Autodesk Inventor part; units mm, degrees
(part 2 of 2)
extrude "Extrusion65" cut sketch "Sketch70" against normal blind 1.5 contours L6 L7 L8 L0 | L4 L17 L14 L15
sketch "Sketch71" plane through (0, 1.5, 0) normal (0, 1, 0) x (1, 0, 0)
  line L0 (6.4642, -4.9) -> (13.4642, -4.9) projected
  line L1 (-3.6078, -4.9) -> (3.3922, -4.9) projected
  line L2 (-3.6078, -3.9) -> (3.3922, -3.9)
  line L3 (6.4642, -3.9) -> (13.4642, -3.9)
  line L4 (-3.4042, -4.9) -> (3.3922, -4.9)
  line L5 (13.4642, -4.9) -> (6.4642, -4.9)
  line L6 (6.4642, -4.9) -> (6.4642, -3.9)
  line L7 (13.4642, -4.9) -> (13.4642, -3.9)
  line L8 (6.4642, -4.9) -> (6.4642, -3.9)
  line L9 (13.4642, -4.9) -> (6.4642, -4.9)
  line L10 (3.3922, -3.9) -> (3.3922, -4.9)
  line L11 (3.3922, -4.9) -> (-3.6078, -4.9)
  line L12 (-3.6078, -4.9) -> (-3.6078, -3.9)
  point P0 (3.3922, -22.9)
  point P1 (0, 0)
  dimension "d349" = 7
  dimension "d351" = 7
  constraints: 22 end point, 4 collinear, 1 point on line
  measures "d349" distance of L2.start L2.end
  measures "d351" distance of L3.start L3.end
extrude "Extrusion66" cut sketch "Sketch71" against normal blind 1.5
sketch "Sketch75" plane through (0, 1.5, 0) normal (0, 1, 0) x (1, 0, 0)
  line L0 (-14, 20) -> (14, 20) projected
  line L1 (-14, 20) -> (0, 20)
  line L2 (0, 20) -> (0, 11.7)
  line L3 (0, 11.7) -> (-11.6, 11.7)
  line L4 (-11.6, 11.7) -> (12, 11.7)
  line L5 (12, 11.7) -> (12, -0.7)
  line L6 (12, -0.7) -> (-11.6, -0.7)
  line L7 (-11.6, -0.7) -> (-11.6, 11.7)
  point P0 (0, 0)
  dimension "d359" = 8.3
  dimension "d360" = 11.6
  dimension "d361" = 23.6
  dimension "d362" = 12.4
  constraints: 14 end point, 3 perpendicular, 2 parallel, 1 horizontal, 1 midpoint
  measures "d359" distance of L1.end L2.end
  measures "d360" distance of L2.end L3.end
  measures "d361" distance of L5.end L6.end
  measures "d362" distance of L4.end L5.end
extrude "Extrusion67" cut sketch "Sketch75" against normal blind 1.5
sketch "Sketch76" plane through (0, 1.5, 0) normal (0, 1, 0) x (1, 0, 0)
  line L0 (-11.6, -0.7) -> (-11.6, 11.7) projected
  circle A0 centre (13.95, 5.5) radius 1.5 projected
  circle A1 centre (-13.95, 5.5) radius 1.5 projected
  line L1 (6.4642, -3.9) -> (13.4642, -3.9) projected
  line L2 (-13.95, 5.5) -> (13.95, 5.5)
  line L3 (-11.6, 11.7) -> (-12, 11.7)
  line L4 (-12, 11.7) -> (-12, -0.7)
  line L5 (-12, -0.7) -> (-11.6, -0.7)
  line L6 (-11.6, 11.7) -> (-11.6, -0.7)
  point P0 (0, 0)
  dimension "d365" = 27.9
  dimension "d366" = 0.4
  constraints: 10 end point, 3 parallel, 2 perpendicular
  measures "d365" distance of L2.start L2.end
  measures "d366" distance of L0.end L3.end
extrude "Extrusion68" cut sketch "Sketch76" against normal blind 1.5 contours L5 L4 L2 L0 | L2 L4 L3 L0
sketch "Sketch77" plane through (0, 1.5, 0) normal (0, 1, 0) x (1, 0, 0)
  line L0 (-12, 11.7) -> (12, 11.7) projected
  line L1 (12, -0.7) -> (-12, -0.7) projected
  line L2 (-12, -0.7) -> (-12, 11.7) projected
  line L3 (-12, 11.7) -> (-12, -0.7)
  line L4 (-12, -0.7) -> (-11.7, -0.7)
  line L5 (-11.7, -0.7) -> (-11.7, 11.7)
  line L6 (-12, 11.7) -> (-11.7, 11.7)
  line L7 (12, 11.7) -> (12, -0.7)
  line L8 (12, -0.7) -> (11.7, -0.7)
  line L9 (11.7, -0.7) -> (11.7, 11.7)
  line L10 (11.7, 11.7) -> (12, 11.7)
  point P0 (0, 0)
  dimension "d370" = 0.3
  dimension "d371" = 0.3
  constraints: 16 end point, 5 perpendicular, 4 point on line, 1 collinear
  measures "d370" distance of L1.end L4.end
  measures "d371" distance of L1.start L8.end
extrude "Extrusion69" add sketch "Sketch77" against normal blind 1.5 contours L0 L5 L1 L2 | L0 L7 L1 L9
sketch "Sketch78" plane through (0, 11.5, 0) normal (0, 1, 0) x (1, 0, 0)
  line L0 (17.5932, -25.4) -> (17.5932, -23.9) projected
  line L1 (17.5932, -23.9) -> (-17.5932, -23.9) projected
  line L2 (-17.5932, -23.9) -> (-17.5932, -25.4) projected
  line L3 (-17.5932, -25.4) -> (17.5932, -25.4) projected
  point P0 (0, 0)
extrude "Extrusion70" cut sketch "Sketch78" against normal blind 10
sketch "Sketch79" plane through (-17.5932, 1.5, 25.4) normal (0, 0, 1) x (1, 0, 0)
  line L0 (35.1864, 0) -> (0, 0) projected
  line L1 (0, -1.5) -> (0, 0) projected
  line L2 (35.1864, -1.5) -> (0, -1.5) projected
  line L3 (35.1864, -1.5) -> (35.1864, 0) projected
  point P0 (17.5932, -1.5)
extrude "Extrusion71" add sketch "Sketch79" along normal blind 10
sketch "Sketch83" plane through (0, 0, 0) normal (0, -1, 0) x (1, 0, 0)
  arc A0 (-26, -4) -> (-17.5932, 11.7729) centre (-36.5932, 11.7729) ccw projected
  arc A1 (17.5932, 11.7729) -> (26, -4) centre (36.5932, 11.7729) ccw projected
  circle A2 centre (-13.95, -5.5) radius 1.5 projected
  circle A3 centre (13.95, -5.5) radius 1.5 projected
  circle A4 centre (12.72, -16.04) radius 1.5 projected
  circle A5 centre (21.72, -4.04) radius 1.5 projected
  circle A6 centre (-21.72, -4.04) radius 1.5 projected
  circle A7 centre (-12.72, -16.04) radius 1.5 projected
  circle A8 centre (-13.95, -5.5) radius 0.1
  circle A9 centre (-21.72, -4.04) radius 0.1
  circle A10 centre (-12.72, -16.04) radius 0.1
  circle A11 centre (12.72, -16.04) radius 0.1
  circle A12 centre (13.95, -5.5) radius 0.1
  circle A13 centre (21.72, -4.04) radius 0.1
  circle A14 centre (-36.5932, 11.7729) radius 0.1
  circle A15 centre (36.5932, 11.7729) radius 0.1
  point P0 (0, 0)
  dimension "d386" = 0.2
  dimension "d387" = 0.2
  dimension "d388" = 0.2
  dimension "d389" = 0.2
  dimension "d390" = 0.2
  dimension "d391" = 0.2
  dimension "d392" = 0.2
  dimension "d393" = 0.2
  constraints: 8 centre point, 8 coincident
  measures "d386" diameter of A8
  measures "d387" diameter of A9
  measures "d388" diameter of A10
  measures "d389" diameter of A11
  measures "d390" diameter of A12
  measures "d391" diameter of A13
  measures "d392" diameter of A14
  measures "d393" diameter of A15
extrude "Extrusion72" add sketch "Sketch83" against normal blind 1.5 contours A2 | A3 | A4 | A5 | A6 | A7
sketch "Sketch84" plane through (0, 0, 0) normal (0, -1, 0) x (1, 0, 0)
  arc A0 (-26, -4) -> (-17.5932, 11.7729) centre (-36.5932, 11.7729) ccw projected
  arc A1 (17.5932, 11.7729) -> (26, -4) centre (36.5932, 11.7729) ccw projected
  circle A2 centre (-36.5932, 11.7729) radius 0.1
  circle A3 centre (36.5932, 11.7729) radius 0.1
  point P0 (0, 0)
  dimension "d396" = 0.2
  dimension "d397" = 0.2
  constraints: 2 centre point, 2 coincident
  measures "d396" diameter of A2
  measures "d397" diameter of A3
extrude "Extrusion73" add sketch "Sketch84" against normal blind 1.5
sketch "Sketch85" plane through (-17.5932, 1.5, 35.4) normal (0, 0, 1) x (1, 0, 0)
  line L0 (35.1864, 0) -> (0, 0) projected
  line L1 (0, 0) -> (0, -1.5) projected
  line L2 (0, -1.5) -> (35.1864, -1.5) projected
  line L3 (35.1864, -1.5) -> (35.1864, 0) projected
  point P0 (17.5932, -1.5)
extrude "Extrusion74" add sketch "Sketch85" along normal blind 0.5
sketch "Sketch86" plane through (0, 0, 0) normal (0, -1, 0) x (1, 0, 0)
  line L0 (-17.5932, 35.9) -> (17.5932, 35.9) projected
  line L1 (11.7, 0.7) -> (11.7, -11.7) projected
  line L2 (0, 35.9) -> (0, 30.9)
  circle A0 centre (0, 30.9) radius 2.5
  point P0 (0, 0)
  dimension "d402" = 5
  dimension "d403" = 5
  constraints: 2 end point, 1 centre point, 1 coincident, 1 midpoint, 1 parallel
  measures "d402" distance of L2.start L2.end
  measures "d403" diameter of A0
extrude "Extrusion75" cut sketch "Sketch86" against normal blind 1.5
sketch "Sketch87" plane through (0, 0, 0) normal (0, -1, 0) x (1, 0, 0)
  line L0 (11.7, 0.7) -> (11.7, -11.7) projected
  line L1 (-0.5745, 30.9) -> (-6.8745, 30.9)
  line L2 (-6.8745, 30.9) -> (5.7255, 30.9)
  circle A0 centre (-6.8745, 30.9) radius 1.5
  circle A1 centre (5.7255, 30.9) radius 1.5
  point P0 (0, 0)
  dimension "d406" = 6.3
  dimension "d407" = 12.6
  dimension "d408" = 3
  dimension "d409" = 3
  constraints: 4 end point, 2 centre point, 2 coincident, 1 perpendicular, 1 point on line
  measures "d406" distance of L1.start L1.end
  measures "d407" distance of L1.end L2.end
  measures "d408" diameter of A0
  measures "d409" diameter of A1
extrude "Extrusion76" cut sketch "Sketch87" against normal blind 1.5
sketch "Sketch88" plane through (0, 0, 0) normal (0, -1, 0) x (1, 0, 0)
  circle A0 centre (-6.8745, 30.9) radius 1.5 projected
  circle A1 centre (5.7255, 30.9) radius 1.5 projected
  circle A2 centre (0, 30.9) radius 2.5 projected
  circle A3 centre (-6.8745, 30.9) radius 0.1
  circle A4 centre (0, 30.9) radius 0.1
  circle A5 centre (5.7255, 30.9) radius 0.1
  point P0 (0, 0)
  dimension "d412" = 0.2
  dimension "d413" = 0.2
  dimension "d414" = 0.2
  constraints: 3 centre point, 3 coincident
  measures "d412" diameter of A3
  measures "d413" diameter of A4
  measures "d414" diameter of A5
extrude "Extrusion77" add sketch "Sketch88" against normal blind 1.5
sketch "Sketch89" plane through (0, 0, 0) normal (0, -1, 0) x (1, 0, 0)
  line L0 (17.5932, 11.7729) -> (17.5932, 35.9) projected
  line L1 (-17.5932, 23.9) -> (17.5932, 23.9)
  line L2 (17.3932, 23.9) -> (-17.5932, 23.9)
  line L3 (17.5932, 23.9) -> (17.5932, 23.91)
  line L4 (17.5932, 23.91) -> (-17.5932, 23.91)
  line L5 (-17.5932, 23.91) -> (-17.5932, 23.9)
  point P0 (0, 0)
  dimension "d421" = 0.01
  constraints: 10 end point, 3 point on line, 2 perpendicular
  measures "d421" distance of L1.end L3.end
extrude "Extrusion78" cut sketch "Sketch89" against normal blind 1.5
sketch "Sketch90" plane through (0, 0, 0) normal (0, -1, 0) x (1, 0, 0)
  line L0 (-17.5932, 23.91) -> (-17.5932, 35.9) projected
  circle A0 centre (0, 30.9) radius 0.1 projected
  line L1 (0, 30.9) -> (-6.3, 30.9)
  line L2 (0, 30.9) -> (6.3, 30.9)
  circle A1 centre (6.3, 30.9) radius 0.1
  circle A2 centre (-6.3, 30.9) radius 0.1
  point P0 (0, 0)
  dimension "d424" = 6.3
  dimension "d425" = 6.3
  dimension "d426" = 0.2
  dimension "d427" = 0.2
  constraints: 4 end point, 2 centre point, 2 coincident, 1 collinear, 1 perpendicular
  measures "d424" distance of L1.start L1.end
  measures "d425" distance of L1.start L2.end
  measures "d426" diameter of A1
  measures "d427" diameter of A2
extrude "Extrusion79" cut sketch "Sketch90" against normal blind 1.5 contours A1 | A2
sketch "Sketch91" plane through (0, 0, 0) normal (0, -1, 0) x (1, 0, 0)
  circle A0 centre (6.3, 30.9) radius 0.1 projected
  circle A1 centre (-6.8745, 30.9) radius 0.1 projected
  point P0 (0, 0)
extrude "Extrusion80" add sketch "Sketch91" against normal blind 1.5
sketch "Sketch92" plane through (0, 0, 0) normal (0, -1, 0) x (1, 0, 0)
  line L0 (-17.5932, 23.91) -> (-17.5932, 35.9) projected
  circle A0 centre (0, 30.9) radius 0.1 projected
  line L1 (0, 30.9) -> (6.3, 30.9)
  circle A1 centre (6.3, 30.9) radius 0.1
  point P0 (0, 0)
  dimension "d432" = 6.3
  dimension "d433" = 0.2
  constraints: 2 end point, 1 centre point, 1 coincident, 1 perpendicular
  measures "d432" distance of L1.start L1.end
  measures "d433" diameter of A1
extrude "Extrusion81" cut sketch "Sketch92" against normal blind 1.5 contours A1
sketch "Sketch93" plane through (0, 0, 0) normal (0, -1, 0) x (1, 0, 0)
  circle A0 centre (5.7255, 30.9) radius 0.1 projected
  point P0 (0, 0)
extrude "Extrusion82" add sketch "Sketch93" against normal blind 1.5
sketch "Sketch94" plane through (0, 0, 0) normal (0, -1, 0) x (1, 0, 0)
  line L0 (-3.6078, 22.9) -> (3.3922, 22.9) projected
  line L1 (3.3922, 22.9) -> (3.3922, 3.9) projected
  line L2 (3.3922, 3.9) -> (-3.6078, 3.9) projected
  line L3 (-0.1078, 22.9) -> (-0.1078, 13.4)
  line L4 (-0.1078, 22.9) -> (-0.1078, 20.9)
  circle A0 centre (-0.1078, 20.9) radius 2
  line L5 (-0.1078, 3.9) -> (-0.1078, 5.9)
  circle A1 centre (-0.1078, 5.9) radius 2
  line L6 (-2.1078, 20.9) -> (-2.1078, 5.9)
  line L7 (1.8922, 20.9) -> (1.8922, 5.9)
  line L8 (-0.1078, 3.9) -> (3.3922, 3.9)
  line L9 (-0.1078, 22.9) -> (3.3922, 22.9)
  line L10 (3.3922, 22.9) -> (3.3922, 3.9)
  line L11 (-3.6078, 22.9) -> (-0.1078, 22.9)
  line L12 (-3.6078, 3.9) -> (-3.6078, 22.9)
  line L13 (-3.6078, 3.9) -> (-0.1078, 3.9)
  arc A2 (1.8922, 20.9) -> (-2.1078, 20.9) centre (-0.1078, 20.9) ccw
  arc A3 (-2.1078, 5.9) -> (1.8922, 5.9) centre (-0.1078, 5.9) ccw
  line L14 (-2.1078, 5.9) -> (-2.1078, 20.9)
  line L15 (1.8922, 20.9) -> (1.8922, 5.9)
  point P0 (0, 0)
  dimension "d438" = 2
  dimension "d439" = 4
  dimension "d441" = 2
  dimension "d442" = 4
  constraints: 26 end point, 11 point on circle, 5 tangent, 4 centre point, 4 collinear, 3 midpoint, 3 perpendicular, 2 coincident, 1 parallel, 1 point on line
  measures "d438" distance of L3.start L4.end
  measures "d439" diameter of A0
  measures "d441" distance of L5.start L5.end
  measures "d442" diameter of A1
extrude "Extrusion83" add sketch "Sketch94" against normal blind 2 contours L0 A0 L6 A1 L2 L12 | L0 L1 L2 A1 L7 A0
sketch "Sketch95" plane through (0, 1.5, 0) normal (0, 1, 0) x (1, 0, 0)
  line L0 (-17.5932, -23.9) -> (17.5932, -23.9) projected
  line L1 (17.5932, -23.9) -> (17.5932, -11.7729) projected
  arc A0 (26, 4) -> (17.5932, -11.7729) centre (36.5932, -11.7729) ccw projected
  line L2 (14, 20) -> (26, 4) projected
  line L3 (-14, 20) -> (14, 20) projected
  line L4 (-26, 4) -> (-14, 20) projected
  arc A1 (-17.5932, -11.7729) -> (-26, 4) centre (-36.5932, -11.7729) ccw projected
  line L5 (-17.5932, -23.9) -> (-17.5932, -11.7729) projected
  circle A2 centre (-21.72, 4.04) radius 0.1 projected
  circle A3 centre (12.72, 16.04) radius 0.1 projected
  circle A4 centre (-13.95, 5.5) radius 0.1 projected
  circle A5 centre (13.95, 5.5) radius 0.1 projected
  circle A6 centre (21.72, 4.04) radius 0.1 projected
  circle A7 centre (-12.72, 16.04) radius 0.1 projected
  line L6 (-11.7, 11.7) -> (11.7, 11.7) projected
  line L7 (11.7, 11.7) -> (11.7, -0.7) projected
  line L8 (11.7, -0.7) -> (-11.7, -0.7) projected
  line L9 (-11.7, -0.7) -> (-11.7, 11.7) projected
  line L10 (-3.6078, -22.9) -> (-3.6078, -3.9) projected
  line L11 (-3.6078, -3.9) -> (-0.1078, -3.9) projected
  line L12 (-0.1078, -3.9) -> (3.3922, -3.9) projected
  line L13 (3.3922, -3.9) -> (3.3922, -22.9) projected
  line L14 (3.3922, -22.9) -> (-0.1078, -22.9) projected
  line L15 (-0.1078, -22.9) -> (-3.6078, -22.9) projected
  line L16 (13.4642, -3.9) -> (13.4642, -22.9) projected
  line L17 (13.4642, -22.9) -> (6.4642, -22.9) projected
  line L18 (6.4642, -22.9) -> (6.4642, -3.9) projected
  line L19 (6.4642, -3.9) -> (13.4642, -3.9) projected
  point P0 (0, 0)
extrude "Extrusion84" add sketch "Sketch95" along normal blind 0.5
sketch "Sketch96" plane through (0, 1.5, 0) normal (0, 1, 0) x (1, 0, 0)
  circle A0 centre (6.3, -30.9) radius 0.1 projected
  circle A1 centre (-6.3, -30.9) radius 0.1 projected
  circle A2 centre (0, -30.9) radius 0.1 projected
  line L0 (17.5932, -23.91) -> (-17.5932, -23.91) projected
  line L1 (-17.5932, -35.9) -> (-17.5932, -23.91) projected
  line L2 (17.5932, -35.9) -> (-17.5932, -35.9) projected
  line L3 (17.5932, -35.9) -> (17.5932, -23.91) projected
  point P0 (0, 0)
extrude "Extrusion85" add sketch "Sketch96" along normal blind 0.5
sketch "Sketch97" plane through (0, 0, 0) normal (0, -1, 0) x (1, 0, 0)
  line L0 (13.4642, 22.9) -> (13.4642, 3.9) projected
  line L1 (13.4642, 3.9) -> (6.4642, 3.9) projected
  line L2 (6.4642, 3.9) -> (6.4642, 22.9) projected
  line L3 (6.4642, 22.9) -> (13.4642, 22.9) projected
  point P0 (0, 0)
extrude "Extrusion86" add sketch "Sketch97" against normal blind 2
sketch "Sketch98" plane through (0, 0, 0) normal (0, -1, 0) x (1, 0, 0)
  arc A0 (-2.1078, 5.9) -> (1.8922, 5.9) centre (-0.1078, 5.9) ccw projected
  line L0 (-2.1078, 5.9) -> (-2.1078, 20.9) projected
  arc A1 (1.8922, 20.9) -> (-2.1078, 20.9) centre (-0.1078, 20.9) ccw projected
  line L1 (1.8922, 20.9) -> (1.8922, 5.9) projected
  line L2 (17.5932, 23.9) -> (-17.5932, 23.9) projected
  line L3 (17.5932, 23.9) -> (13.0932, 23.9)
  line L4 (13.0932, 23.9) -> (13.0932, 20.9)
  line L5 (-17.5932, 23.9) -> (-13.0932, 23.9)
  line L6 (-13.0932, 23.9) -> (-13.0932, 20.9)
  line L7 (11.5932, 20.9) -> (11.5932, 5.9)
  line L8 (14.5932, 20.9) -> (14.5932, 5.9)
  line L9 (-14.5932, 20.9) -> (-14.5932, 5.9)
  line L10 (-11.5932, 20.9) -> (-11.5932, 5.9)
  circle A2 centre (-13.0932, 20.9) radius 0.1
  circle A3 centre (-13.0932, 5.9) radius 0.1
  circle A4 centre (13.0932, 20.9) radius 0.1
  circle A5 centre (13.0932, 5.9) radius 0.1
  line L11 (11.5932, 5.9) -> (14.5932, 5.9)
  line L12 (11.5932, 20.9) -> (14.5932, 20.9)
  line L13 (-14.5932, 20.9) -> (-11.5932, 20.9)
  line L14 (-14.5932, 5.9) -> (-11.5932, 5.9)
  circle A6 centre (-0.1078, 20.9) radius 0.1
  circle A7 centre (-0.1078, 5.9) radius 0.1
  point P0 (0, 0)
  dimension "d451" = 4.5
  dimension "d452" = 3
  dimension "d453" = 4.5
  dimension "d454" = 3
  dimension "d459" = 0.2
  dimension "d460" = 0.2
  dimension "d461" = 0.2
  dimension "d462" = 0.2
  dimension "d463" = 0.2
  dimension "d464" = 0.2
  constraints: 24 end point, 6 centre point, 3 parallel, 3 perpendicular, 2 coincident, 2 point on line
  measures "d451" distance of L2.start L3.end
  measures "d452" distance of L3.end L4.end
  measures "d453" distance of L2.end L5.end
  measures "d454" distance of L5.end L6.end
  measures "d459" diameter of A2
  measures "d460" diameter of A3
  measures "d461" diameter of A4
  measures "d462" diameter of A5
  measures "d463" diameter of A6
  measures "d464" diameter of A7
extrude "Extrusion87" cut sketch "Sketch98" against normal blind 2 contours L0 A1 L1 A0 | A4 L12 L4 | L4 L12 A4 | L12 A4 | L11 A5 | A5 L11 | A2 L13 L6 | L6 L13 A2 | L13 A2 | L14 A3 | A3 L14
sketch "Sketch99" plane through (0, 0, 0) normal (0, -1, 0) x (1, 0, 0)
  arc A0 (-2.1078, 5.9) -> (1.8922, 5.9) centre (-0.1078, 5.9) ccw projected
  line L0 (-2.1078, 5.9) -> (-2.1078, 20.9) projected
  arc A1 (1.8922, 20.9) -> (-2.1078, 20.9) centre (-0.1078, 20.9) ccw projected
  line L1 (1.8922, 20.9) -> (1.8922, 5.9) projected
  circle A2 centre (-0.1078, 5.9) radius 0.1
  circle A3 centre (-0.1078, 20.9) radius 0.1
  point P0 (0, 0)
  dimension "d467" = 0.2
  dimension "d468" = 0.2
  constraints: 2 centre point, 2 coincident
  measures "d467" diameter of A2
  measures "d468" diameter of A3
extrude "Extrusion88" add sketch "Sketch99" against normal blind 2
sketch "Sketch100" plane through (0, 0, 0) normal (0, -1, 0) x (1, 0, 0)
  circle A0 centre (-0.1078, 5.9) radius 0.1 projected
  circle A1 centre (-0.1078, 20.9) radius 0.1 projected
  circle A2 centre (13.0932, 5.9) radius 0.1 projected
  circle A3 centre (-13.0932, 5.9) radius 0.1 projected
  circle A4 centre (-13.0932, 20.9) radius 0.1 projected
  circle A5 centre (13.0932, 20.9) radius 0.1 projected
  line L0 (17.5932, 11.7729) -> (17.5932, 23.9) projected
  line L1 (-13.0932, 20.9) -> (-13.0932, 5.9)
  line L2 (-0.1078, 20.9) -> (-0.1078, 5.9)
  line L3 (13.0932, 20.9) -> (13.0932, 5.9)
  line L4 (-14.5932, 6.15) -> (-11.5932, 6.15)
  line L5 (-11.5932, 6.15) -> (-11.5932, 20.65)
  line L6 (-11.5932, 20.65) -> (-14.5932, 20.65)
  line L7 (-14.5932, 20.65) -> (-14.5932, 6.15)
  line L8 (-14.5932, 6.15) -> (-11.5932, 20.65) construction
  line L9 (-11.5932, 6.15) -> (-14.5932, 20.65) construction
  line L10 (1.8922, 20.65) -> (-2.1078, 20.65)
  line L11 (-2.1078, 20.65) -> (-2.1078, 6.15)
  line L12 (-2.1078, 6.15) -> (1.8922, 6.15)
  line L13 (1.8922, 6.15) -> (1.8922, 20.65)
  line L14 (1.8922, 20.65) -> (-2.1078, 6.15) construction
  line L15 (-2.1078, 20.65) -> (1.8922, 6.15) construction
  line L16 (11.5932, 20.65) -> (14.5932, 20.65)
  line L17 (14.5932, 20.65) -> (14.5932, 6.15)
  line L18 (14.5932, 6.15) -> (11.5932, 6.15)
  line L19 (11.5932, 6.15) -> (11.5932, 20.65)
  line L20 (11.5932, 20.65) -> (14.5932, 6.15) construction
  line L21 (14.5932, 20.65) -> (11.5932, 6.15) construction
  point P0 (0, 0)
  point P1 (-13.0932, 13.4)
  point P2 (-0.1078, 13.4)
  point P3 (13.0932, 13.4)
  dimension "d471" = 3
  dimension "d472" = 14.5
  dimension "d473" = 4
  dimension "d474" = 14.5
  dimension "d475" = 3
  dimension "d476" = 14.5
  constraints: 42 end point, 9 midpoint, 9 parallel, 3 horizontal, 3 perpendicular
  measures "d471" distance of L6.end L5.end
  measures "d472" distance of L5.end L4.end
  measures "d473" distance of L12.end L11.end
  measures "d474" distance of L11.end L10.end
  measures "d475" distance of L17.end L18.end
  measures "d476" distance of L16.end L17.end
extrude "Extrusion89" cut sketch "Sketch100" against normal blind 2 contours L6 L5 L4 L1 | L1 L4 L7 L6 | L10 L13 L12 L2 | L2 L12 L11 L10 | L16 L17 L18 L3 | L3 L18 L19 L16
sketch "Sketch101" plane through (0, 0, 0) normal (0, -1, 0) x (1, 0, 0)
  line L0 (-2.1078, 6.15) -> (-2.1078, 20.65) projected
  line L1 (-2.1078, 20.65) -> (1.8922, 20.65) projected
  line L2 (1.8922, 20.65) -> (1.8922, 6.15) projected
  line L3 (1.8922, 6.15) -> (-2.1078, 6.15) projected
  circle A0 centre (-0.1078, 5.9) radius 0.1 projected
  circle A1 centre (-0.1078, 20.9) radius 0.1 projected
  point P0 (0, 0)
extrude "Extrusion90" add sketch "Sketch101" against normal blind 2
sketch "Sketch102" plane through (0, 0, 0) normal (0, -1, 0) x (1, 0, 0)
  line L0 (11.5932, 20.65) -> (14.5932, 20.65) projected
  circle A0 centre (0, 20.9) radius 0.1
  circle A1 centre (0, 5.9) radius 0.1
  line L1 (0, 20.9) -> (0, 5.9)
  line L2 (2, 20.65) -> (-2, 20.65)
  line L3 (-2, 20.65) -> (-2, 6.15)
  line L4 (-2, 6.15) -> (2, 6.15)
  line L5 (2, 6.15) -> (2, 20.65)
  line L6 (2, 20.65) -> (-2, 6.15) construction
  line L7 (-2, 20.65) -> (2, 6.15) construction
  point P0 (0, 0)
  point P1 (0, 13.4)
  dimension "d481" = 0.2
  dimension "d482" = 0.2
  dimension "d483" = 4
  dimension "d484" = 14.5
  constraints: 14 end point, 3 midpoint, 2 centre point, 2 parallel, 2 perpendicular, 1 horizontal
  measures "d481" diameter of A0
  measures "d482" diameter of A1
  measures "d483" distance of L4.end L3.end
  measures "d484" distance of L3.end L2.end
extrude "Extrusion91" cut sketch "Sketch102" against normal blind 2
body "Solid1"
